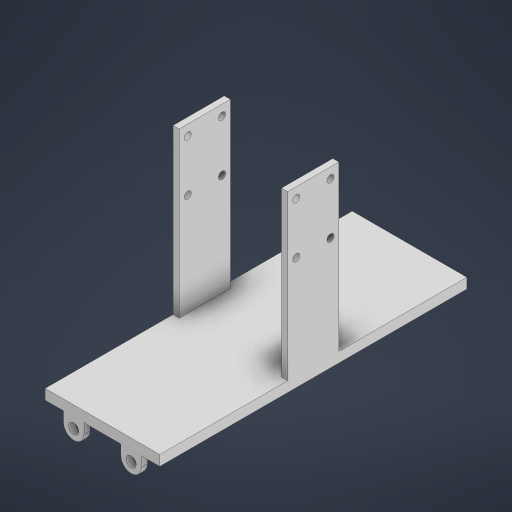
# Autodesk Inventor part: Mounting atas
Saved by Autodesk Inventor 2023.6 (Build 276521000, 521)
## iProperties
Created: 2026-03-05
Part Number: Mounting atas
Material: Generic
Document SubType Name: Modeling
Designer: user
Density: 1 g/cm^3
Appearance: Default
Author: user
Autodesk Inventor part; units mm, degrees
ref_plane "YZ Plane" through (0, 0, 0) normal (1, 0, 0) x (0, 1, 0)
ref_plane "XZ Plane" through (0, 0, 0) normal (0, 1, 0) x (-1, 0, 0)
sketch "Sketch1" plane through (0, 0, 0) normal (0, 1, 0) x (-1, 0, 0)
  line L0 (28, 75) -> (-28, 75)
  line L1 (-28, 75) -> (-28, -75)
  line L2 (-28, -75) -> (28, -75)
  line L3 (28, -75) -> (28, 75)
  line L4 (28, 75) -> (-28, -75) construction
  line L5 (-28, 75) -> (28, -75) construction
  point P0 (0, 0)
  dimension "d0" = 56
  dimension "d1" = 150
  constraints: 12 end point, 2 midpoint, 2 parallel, 1 horizontal, 1 perpendicular
  measures "d0" distance between parallel lines of L1 L3
  measures "d1" distance between parallel lines of L2 L0
extrude "Extrusion1" add sketch "Sketch1" along normal blind 5
sketch "Sketch2" plane through (0, 5, 0) normal (0, 1, 0) x (1, 0, 0)
  line L0 (-28, 12.5) -> (-25, 12.5)
  line L1 (-25, 12.5) -> (-25, -12.5)
  line L2 (-25, -12.5) -> (-28, -12.5)
  line L3 (-28, -12.5) -> (-28, 12.5)
  line L4 (-28, 75) -> (-28, -75) projected
  line L5 (0, 0) -> (0, 30.0888)
  line L6 (28, 12.5) -> (25, 12.5)
  line L7 (25, 12.5) -> (25, -12.5)
  line L8 (25, -12.5) -> (28, -12.5)
  line L9 (28, -12.5) -> (28, 12.5)
  point P0 (-28, 0)
  dimension "d4" = 3
  dimension "d5" = 25
  constraints: 18 end point, 4 symmetric about line, 2 midpoint, 2 parallel, 1 horizontal, 1 perpendicular, 1 vertical
  measures "d4" distance between parallel lines of L1 L3
  measures "d5" distance between parallel lines of L0 L2
extrude "Extrusion2" add sketch "Sketch2" along normal blind 80
sketch "Sketch3" plane through (28, 0, 75) normal (1, 0, 0) x (0, 0, -1)
  circle A0 centre (66.65, 55) radius 1.75
  circle A1 centre (66.65, 80) radius 1.75
  circle A2 centre (83.35, 80) radius 1.75
  circle A3 centre (83.35, 55) radius 1.75
  circle A4 centre (66.65, 55) radius 1.75
  circle A5 centre (66.65, 80) radius 1.75
  circle A6 centre (83.35, 80) radius 1.75
  circle A7 centre (83.35, 55) radius 1.75
  line L0 (83.35, 55) -> (66.65, 80)
  line L1 (66.65, 80) -> (66.65, 55)
  line L2 (66.65, 55) -> (83.35, 80)
  line L3 (83.35, 80) -> (83.35, 55)
  line L4 (66.65, 55) -> (83.35, 55)
  line L5 (83.35, 80) -> (66.65, 80)
  line L6 (0, 0) -> (150, 0) projected
  line L7 (150, 0) -> (150, 5) projected
  line L8 (87.5, 5) -> (150, 5) projected
  line L9 (87.5, 5) -> (87.5, 85) projected
  line L10 (62.5, 85) -> (87.5, 85) projected
  line L11 (62.5, 5) -> (62.5, 85) projected
  line L12 (0, 5) -> (62.5, 5) projected
  line L13 (0, 0) -> (0, 5) projected
  line L14 (62.5, 80) -> (87.5, 80)
  line L15 (87.5, 5) -> (87.5, 85) projected
  point P0 (75, 0)
  point P1 (75, 80)
  dimension "d12" = 5
  dimension "d14" = 16.7
  dimension "d15" = 25
  constraints: 14 end point, 8 centre point, 4 coincident, 4 concentric, 2 midpoint, 2 parallel, 2 point on line, 1 perpendicular, 1 vertical
  measures "d12" distance between parallel lines of L10 L14
  measures "d14" distance between parallel lines of L3 L1
  measures "d15" distance of L0.end L1.end
extrude "Extrusion3" cut sketch "Sketch3" against normal through all contours L4 L2 A0 | A0 L1 L4 | L2 L1 A0 | L4 L3 A3 | A3 L0 L4 | L1 L0 A1 | A1 L14 L1 | A3 L3 L0 | L0 L5 A1 | L2 L3 A2 | A2 L5 L2 | A1 L5 L14 | A2 L14 L5 | L3 L14 A2
sketch "Sketch4" plane through (-28, 0, 75) normal (0, 0, 1) x (1, 0, 0)
  circle A0 centre (14, 10) radius 2.5
  circle A1 centre (42, 10) radius 2.5
  line L0 (6.5, 5) -> (9, 5)
  line L1 (47, 5) -> (49.5, 5)
  line L2 (47, 10) -> (47, 5)
  arc A2 (47, 10) -> (37, 10) centre (42, 10) ccw
  line L3 (37, 5) -> (37, 10)
  line L4 (19, 5) -> (37, 5)
  line L5 (19, 10) -> (19, 5)
  arc A3 (19, 10) -> (9, 10) centre (14, 10) ccw
  line L6 (9, 5) -> (9, 10)
  line L7 (0, 5) -> (56, 5) projected
  point P0 (28, 0)
  point P1 (33.2021, 4.5034)
  point P2 (28, 5)
  point P3 (9, 5)
  dimension "d18" = 43
  dimension "d19" = 18
  dimension "d20" = 5
  dimension "d21" = 5
  dimension "d22" = 5
  dimension "d23" = 5
  dimension "d24" = 5
  dimension "d25" = 5
  constraints: 14 end point, 4 centre point, 4 point on circle, 2 coincident, 2 midpoint
  measures "d18" distance of L1.end L0.start
  measures "d19" distance of L4.start L3.start
  measures "d20" diameter of A0
  measures "d21" radius of A3
  measures "d22" radius of A2
  measures "d23" diameter of A1
  measures "d24" distance of L5.start L4.start
  measures "d25" distance of L3.start L3.end
extrude "Extrusion4" add sketch "Sketch4" against normal blind 3
ref_plane "Work Plane1" through (0, 2.5, 0) normal (0, -1, 0) x (1, 0, 0)
mirror "Mirror1" about plane through (0, 2.5, 0) normal (0, -1, 0) of "Extrusion4"
mirror "Mirror2" about plane through (0, 0, 0) normal (0, 0, 1) of "Extrusion4", "Mirror1"
sketch "Sketch5" plane through (28, 0, 75) normal (0, 0, 1) x (1, 0, 0)
  line L0 (-47, 5) -> (-56, 5) projected
  line L1 (0, 5) -> (-9, 5) projected
  line L2 (-47, 5) -> (-9, 5)
  circle A0 centre (-14, -5) radius 2.5 projected
  circle A1 centre (-42, -5) radius 2.5 projected
  circle A2 centre (-14, 10) radius 2.5 projected
  circle A3 centre (-42, 10) radius 2.5 projected
  line L3 (-56, 0) -> (-47, 0) projected
  line L4 (-47, -5) -> (-47, 0) projected
  arc A4 (-47, -5) -> (-37, -5) centre (-42, -5) ccw projected
  line L5 (-37, 0) -> (-37, -5) projected
  line L6 (-37, 0) -> (-19, 0) projected
  line L7 (-19, -5) -> (-19, 0) projected
  arc A5 (-19, -5) -> (-9, -5) centre (-14, -5) ccw projected
  line L8 (-9, 0) -> (-9, -5) projected
  line L9 (-9, 0) -> (0, 0) projected
  line L10 (0, 0) -> (0, 5) projected
  line L11 (-9, 5) -> (0, 5) projected
  line L12 (-9, 5) -> (-9, 10) projected
  arc A6 (-9, 10) -> (-19, 10) centre (-14, 10) ccw projected
  line L13 (-19, 10) -> (-19, 5) projected
  line L14 (-37, 5) -> (-19, 5) projected
  line L15 (-37, 5) -> (-37, 10) projected
  arc A7 (-37, 10) -> (-47, 10) centre (-42, 10) ccw projected
  line L16 (-47, 10) -> (-47, 5) projected
  line L17 (-56, 5) -> (-47, 5) projected
  line L18 (-56, 0) -> (-56, 5) projected
  point P0 (-28, 0)
  constraints: 2 end point, 1 horizontal
extrude "Extrusion5" cut sketch "Sketch5" against normal through all contours L16 A7 L15 L2 | L13 A6 L12 L2
body "Solid1"
